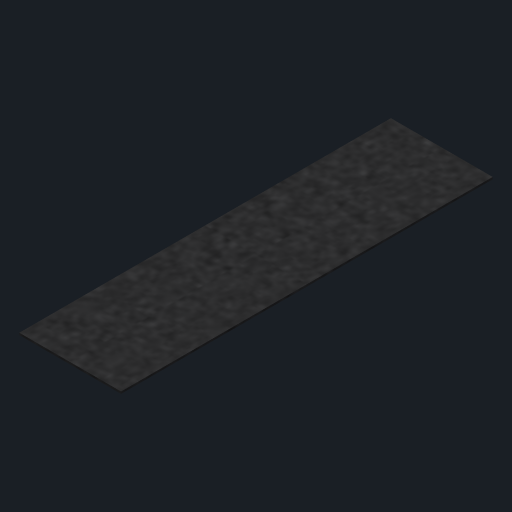
# Autodesk Inventor part: DESLIZANTE
Saved by Autodesk Inventor 2024.3 (Build 283343000, 343)
## iProperties
Created: 2024-08-24
Part Number: DESLIZANTE
Material: Steel, Mild, Welded
Document SubType Name: Modeling
Designer: Niler
Density: 7.85 g/cm^3
Appearance: Weld - Steel Mild
Author: Niler
Autodesk Inventor part; units mm, degrees
ref_plane "YZ Plane" through (0, 0, 0) normal (1, 0, 0) x (0, 1, 0)
ref_plane "XZ Plane" through (0, 0, 0) normal (0, 1, 0) x (-1, 0, 0)
ref_plane "XY Plane" through (0, 0, 0) normal (0, 0, 1) x (1, 0, 0)
sketch "Sketch1" plane through (0, 0, 0) normal (0, 1, 0) x (-1, 0, 0)
  line L0 (-50, 182.5) -> (50, 182.5)
  line L1 (50, 182.5) -> (50, -182.5)
  line L2 (50, -182.5) -> (-50, -182.5)
  line L3 (-50, -182.5) -> (-50, 182.5)
  line L4 (-50, 182.5) -> (50, -182.5) construction
  line L5 (50, 182.5) -> (-50, -182.5) construction
  point P0 (0, 0)
  dimension "d0" = 100
  dimension "d1" = 365
  constraints: 12 end point, 2 midpoint, 2 parallel, 1 horizontal, 1 perpendicular
  measures "d0" distance of L1.end L2.end
  measures "d1" distance of L0.end L1.end
extrude "Extrusion1" add sketch "Sketch1" along normal blind 2
body "Solid1"
